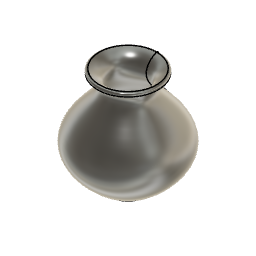
vase_model (Autodesk Fusion 360 design; units mm, degrees)
Autodesk Fusion 360 part; units mm, degrees
sketch "Sketch1" plane through (0, 0, 0) normal (0, 0, 1) x (1, 0, 0)
  line L0 (-50, 50) -> (50, 50)
  line L1 (50, 50) -> (50, -50)
  line L2 (50, -50) -> (-50, -50)
  line L3 (-50, -50) -> (-50, 50)
  line L4 (-50, 50) -> (50, -50) construction
  line L5 (50, 50) -> (-50, -50) construction
  constraint perpendicular L0 L1
  constraint parallel L0 L2
  constraint parallel L1 L3
  constraint horizontal L0
  constraint coincident L4 origin
  constraint coincident L5 origin
sketch "Sketch2" plane through (0, 0, 100) normal (0, 0, 1) x (-1, 0, 0)
sketch "Sketch3" plane through (0, 0, 100) normal (0, 0, 1) x (-1, 0, 0)
sketch "Sketch4" plane through (0, 0, 0) normal (1, 0, 0) x (0, 1, 0)
  spline S0 degree 5 poles (54.2185, 125.1155) (51.8513, 123.9321) (47.5961, 121.462) (42.6512, 117.4472) (38.9561, 111.4702) (39.1161, 102.9461) (43.7062, 93.3754) (51.7839, 82.8153) (61.9213, 71.3664) (72.4574, 59.1504) (81.6949, 46.2966) (88.0974, 32.9282) (90.5324, 19.1499) (88.3812, 5.0405) (81.3542, -9.3423) (69.3905, -23.9603) (55.9163, -35.8244) (43.6569, -44.8132) (34.5336, -50.8458) (29.7343, -53.8721) knots 0 0 0 0 0 0 0.066667 0.133333 0.2 0.266667 0.333333 0.4 0.466667 0.533333 0.6 0.666667 0.733333 0.8 0.866667 0.933333 1 1 1 1 1 1
  spline S1 degree 3 poles (51.1092, 131.3351) (46.6438, 129.1027) (42.8577, 126.579) (39.8125, 123.5465) (37.2632, 121.0078) (35.2405, 118.0715) (34.017, 114.808) (32.8369, 111.6599) (32.4462, 108.2558) (32.7703, 104.9491) (33.1744, 100.8272) (34.6081, 96.8743) (36.6194, 93.0327) (39.5984, 87.3428) (43.8893, 81.7849) (48.6869, 76.0474) (54.984, 68.5166) (62.1616, 60.6989) (68.1517, 52.7571) (72.4862, 47.0104) (76.1687, 41.2222) (78.6499, 35.5463) (81.2159, 29.6764) (82.5189, 23.9667) (82.4322, 18.2079) (82.3468, 12.5298) (80.9266, 6.7257) (77.8465, 0.5454) (74.0998, -6.9726) (67.842, -15.0022) (58.9182, -23.3287) (50.3486, -31.3246) (39.3597, -39.582) (26.0254, -47.9903) knots 0 0 0 0 0.067262 0.067262 0.067262 0.123571 0.123571 0.123571 0.177889 0.177889 0.177889 0.245597 0.245597 0.245597 0.345883 0.345883 0.345883 0.477516 0.477516 0.477516 0.572767 0.572767 0.572767 0.671272 0.671272 0.671272 0.768399 0.768399 0.768399 0.886545 0.886545 0.886545 1 1 1 1
  spline S2 degree 5 poles (51.1092, 131.3351) (51.3245, 131.3051) (51.7416, 131.2368) (52.3268, 131.1093) (53.0246, 130.8885) (53.7502, 130.5222) (54.3167, 130.0578) (54.7118, 129.4877) (54.9301, 128.8087) (54.9804, 128.026) (54.8758, 127.148) (54.6789, 126.3756) (54.4715, 125.7596) (54.3072, 125.3329) (54.2185, 125.1155) knots 0 0 0 0 0 0 0.1 0.2 0.3 0.4 0.5 0.6 0.7 0.8 0.9 1 1 1 1 1 1
  line L0 (29.7343, -53.8721) -> (0, -53.8721)
  line L1 (26.0254, -47.9903) -> (0, -47.9903)
  line L2 (0, -47.9903) -> (0, -53.8721)
  point P0 (41.0782, 100)
  point P1 (85.4569, 37.3103)
  point P2 (54.6322, 129.53)
  dimension "d12" = 6.9535
  constraint horizontal L0
  constraint horizontal L1
  constraint perpendicular L0 L2
revolve "Revolve2" add sketch "Sketch4" angle 360 about axis through (0, 0, 1.75) along (0, 0, 1)
revolve "Revolve1" [suppressed]
